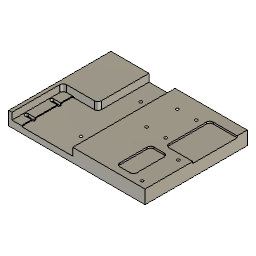
x_stage (Autodesk Fusion 360 design; units mm, degrees)
part number: 2025-09-14-11-39-11-574
Autodesk Fusion 360 part; units mm, degrees
sketch "Sketch1" plane through (0, 0, 0) normal (0, 0, 1) x (1, 0, 0)
  line L0 (-50, 50) -> (50, 50)
  line L1 (50, 50) -> (50, -50)
  line L2 (50, -50) -> (-50, -50)
  line L3 (-50, -50) -> (-50, 50)
  line L4 (-50, 50) -> (50, -50) construction
  line L5 (50, 50) -> (-50, -50) construction
  circle A0 centre (-37.5, 37.5) radius 3.125
  circle A1 centre (-37.5, -37.5) radius 3.125
  circle A2 centre (37.5, -37.5) radius 3.125
  circle A3 centre (37.5, 37.5) radius 3.125
  dimension "d1" = 100
  dimension "d2" = 100
  dimension "d5" = 6.25
  dimension "d6" = 75
  dimension "d7" = 75
  constraint horizontal L0
  constraint perpendicular L0 L1
  constraint parallel L0 L2
  constraint parallel L1 L3
  constraint coincident L4 origin
  constraint coincident L5 origin
  constraint vertical A2.centre A3.centre
  constraint horizontal A0.centre A3.centre
  constraint vertical A0.centre A1.centre
  constraint horizontal A1.centre A2.centre
  constraint equal A2 A3
  constraint equal A1 A2
  constraint equal A0 A1
  constraint coincident L5 A1.centre
  constraint coincident L4 A0.centre
  measures "d1" distance of L0.start L0.end
  measures "d2" distance of L0.start L2.end
  measures "d5" diameter of A0
  measures "d6" distance of A0.centre A3.centre
  measures "d7" distance of A0.centre A1.centre
extrude "Extrude2" add sketch "Sketch1" along normal blind 8
sketch "Sketch2" plane through (0, 0, 8) normal (0, 0, 1) x (-1, 0, 0)
  circle A0 centre (-37.5, -37.5) radius 3.125
  circle A1 centre (37.5, -37.5) radius 3.125
  circle A2 centre (-37.5, 37.5) radius 3.125
  circle A3 centre (37.5, 37.5) radius 3.125
  line L0 (50, 50) -> (-50, 50)
  line L1 (-50, 50) -> (-50, -50)
  line L2 (-50, -50) -> (50, -50)
  line L3 (50, -50) -> (50, 50)
  line L4 (30, -30) -> (-30, -30) construction
  line L5 (-30, -30) -> (-30, 30) construction
  line L6 (-30, 30) -> (30, 30) construction
  line L7 (30, 30) -> (30, -30) construction
  line L8 (30, -30) -> (-30, 30) construction
  line L9 (-30, -30) -> (30, 30) construction
  line L10 (-7.6, -41) -> (7.6, -41)
  line L11 (7.6, -41) -> (7.6, 41)
  line L12 (7.6, 41) -> (-7.6, 41)
  line L13 (-7.6, 41) -> (-7.6, -41)
  line L14 (7.6, 30) -> (28, 30)
  line L15 (28, 30) -> (28, 0)
  line L16 (28, 0) -> (7.6, 0)
  line L17 (7.6, 0) -> (7.6, 30)
  line L18 (28, 30) -> (22.5, 30)
  line L19 (22.5, 30) -> (22.5, 50)
  line L20 (22.5, 50) -> (28, 50)
  line L21 (28, 50) -> (28, 30)
  dimension "d12" = 60
  dimension "d13" = 60
  dimension "d14" = 22.4
  dimension "d15" = 15.2
  dimension "d16" = 11
  dimension "d17" = 11
  dimension "d18" = 30
  dimension "d19" = 20.4
  dimension "d20" = 5.5
  constraint horizontal L4
  constraint perpendicular L4 L5
  constraint parallel L4 L6
  constraint parallel L5 L7
  constraint coincident L8 origin
  constraint coincident L9 origin
  constraint horizontal L10
  constraint vertical L11
  constraint horizontal L12
  constraint vertical L13
  constraint horizontal L14
  constraint vertical L15
  constraint horizontal L16
  constraint vertical L17
  constraint coincident L11 L14.start
  constraint coincident L6 L14.start
  constraint horizontal L18
  constraint vertical L19
  constraint horizontal L20
  constraint vertical L21
  constraint coincident L0 L19.end
  measures "d12" distance of L4.start L4.end
  measures "d13" distance of L4.start L6.end
  measures "d14" distance of L5 L13
  measures "d15" distance of L10.start L10.end
  measures "d16" distance of L4 L10
  measures "d17" distance of L6 L12
  measures "d18" distance of L14.end L15.end
  measures "d19" distance of L15.end L16.end
  measures "d20" distance of L19 L21
extrude "Extrude3" cut sketch "Sketch2" against normal blind 4.5 contours L0 L14 L18 L19 L20 L21 | L11 L14 L15 L16 L17 L18 | L10 L11 L12 L13 L17
fillet "Fillet1" radius 2 7 edges at (-7.6, -30, 5.75) (-7.6, -41, 5.75) (7.6, -41, 5.75) (7.6, 41, 5.75) (-7.6, 41, 5.75) (-7.6, 0, 5.75) (-28, 0, 5.75)
sketch "Sketch3" plane through (0, 0, 8) normal (0, 0, 1) x (-1, 0, 0)
  circle A0 centre (37.5, 37.5) radius 3.125
  circle A1 centre (-37.5, 37.5) radius 3.125
  circle A2 centre (37.5, -37.5) radius 3.125
  circle A3 centre (-37.5, -37.5) radius 3.125
  line L0 (22.5, 30) -> (22.5, 50)
  line L1 (22.5, 50) -> (-50, 50)
  line L2 (-50, 50) -> (-50, -50)
  line L3 (50, -50) -> (50, 50)
  line L4 (50, 50) -> (28, 50)
  line L5 (28, 50) -> (28, 2)
  arc A4 (26, 0) -> (28, 2) centre (26, 2) ccw
  line L6 (26, 0) -> (9.6, 0)
  arc A5 (9.6, 0) -> (7.6, -2) centre (9.6, -2) ccw
  line L7 (7.6, -2) -> (7.6, -39)
  arc A6 (5.6, -41) -> (7.6, -39) centre (5.6, -39) ccw
  arc A7 (-5.6, 41) -> (-7.6, 39) centre (-5.6, 39) ccw
  line L8 (-5.6, 41) -> (5.6, 41)
  arc A8 (7.6, 39) -> (5.6, 41) centre (5.6, 39) ccw
  line L9 (7.6, 39) -> (7.6, 32)
  arc A9 (7.6, 32) -> (9.6, 30) centre (9.6, 32) ccw
  line L10 (9.6, 30) -> (22.5, 30)
  circle A10 centre (0, -17.5) radius 1.5
  circle A11 centre (0, 17.5) radius 1.5
  circle A12 centre (-19, -2) radius 1.5
  circle A13 centre (-30, -2) radius 1.5
  circle A14 centre (-30, -20) radius 1.5
  circle A15 centre (-19, -20) radius 1.5
  line L11 (26.5, 9) -> (22.5, 9)
  arc A16 (22.5, 9) -> (22.5, 7) centre (22.5, 8) ccw
  line L12 (22.5, 7) -> (26.5, 7)
  arc A17 (26.5, 7) -> (26.5, 9) centre (26.5, 8) ccw
  line L13 (26.5, 8) -> (22.5, 8) construction
  line L14 (26.5, 24) -> (22.5, 24)
  arc A18 (22.5, 24) -> (22.5, 22) centre (22.5, 23) ccw
  line L15 (22.5, 22) -> (26.5, 22)
  arc A19 (26.5, 22) -> (26.5, 24) centre (26.5, 23) ccw
  line L16 (26.5, 23) -> (22.5, 23) construction
  line L17 (-30, -30) -> (-30, 30)
  line L18 (30, -30) -> (-30, -30)
  line L19 (30, 30) -> (30, -30)
  line L20 (-30, 30) -> (30, 30)
  circle A20 centre (-45, 5.5) radius 1.5
  circle A21 centre (-45, 26.7) radius 1.5
  line L21 (-50, -50) -> (50, -50)
  line L22 (-7.6, -39) -> (-7.6, 39)
  dimension "d27" = 3
  dimension "d28" = 3
  dimension "d29" = 1
  dimension "d30" = 4
  dimension "d32" = 15
  dimension "d33" = 7
  dimension "d34" = 35
  dimension "d35" = 17.5
  dimension "d36" = 11
  dimension "d37" = 18
  dimension "d43" = 30
  dimension "d48" = 7.5
  dimension "d94" = 21.2
  dimension "d95" = 3
  dimension "d96" = 100
  dimension "d98" = 5
  dimension "d122" = 30
  dimension "d123" = 7.5
  dimension "d141" = 69
  constraint tangent L11 A16
  constraint tangent A16 L12
  constraint parallel L11 L12
  constraint tangent L12 A17
  constraint tangent L11 A17
  constraint horizontal L13
  constraint tangent L14 A18
  constraint tangent A18 L15
  constraint parallel L14 L15
  constraint tangent L15 A19
  constraint tangent L14 A19
  constraint horizontal L16
  constraint equal A10 A11
  constraint equal A12 A13
  constraint equal A12 A15
  constraint equal A14 A15
  constraint horizontal A14.centre A15.centre
  constraint vertical A13.centre A14.centre
  constraint horizontal A12.centre A13.centre
  constraint vertical A12.centre A15.centre
  constraint vertical A10.centre A11.centre
  constraint vertical A16.centre A18.centre
  constraint vertical A17.centre A19.centre
  constraint equal A16 A18
  constraint vertical origin A11.centre
  constraint vertical A20.centre A21.centre
  constraint equal A20 A21
  measures "d27" diameter of A11
  measures "d28" diameter of A12
  measures "d29" radius of A17
  measures "d30" distance of A18.end L15.end
  measures "d32" distance of A17.centre A19.centre
  measures "d33" distance of L10 A18.centre
  measures "d34" distance of A10.centre A11.centre
  measures "d35" distance of origin A10.centre
  measures "d36" distance of A12.centre A13.centre
  measures "d37" distance of A12.centre A15.centre
  measures "d43" distance of L6 L18
  measures "d48" distance of A16.centre L19
  measures "d94" distance of A20.centre A21.centre
  measures "d95" diameter of A20
  measures "d96" distance of L3.start L3.end
  measures "d98" distance of L2 A20.centre
  measures "d122" distance of A14.centre L21
  measures "d123" vertical distance of A13.centre A20.centre
  measures "d141" distance of L3 A15.centre
sketch "Sketch4" plane through (0, 0, 3.5) normal (0, 0, 1) x (-1, 0, 0)
  arc A0 (5.6, -41) -> (7.6, -39) centre (5.6, -39) ccw
  line L0 (7.6, -39) -> (7.6, -2)
  arc A1 (9.6, 0) -> (7.6, -2) centre (9.6, -2) ccw
  line L1 (9.6, 0) -> (26, 0)
  arc A2 (26, 0) -> (28, 2) centre (26, 2) ccw
  line L2 (28, 2) -> (28, 50)
  line L3 (28, 50) -> (22.5, 50)
  line L4 (22.5, 50) -> (22.5, 30)
  line L5 (22.5, 30) -> (9.6, 30)
  arc A3 (7.6, 32) -> (9.6, 30) centre (9.6, 32) ccw
  line L6 (7.6, 32) -> (7.6, 39)
  arc A4 (7.6, 39) -> (5.6, 41) centre (5.6, 39) ccw
  line L7 (5.6, 41) -> (-5.6, 41)
  arc A5 (-5.6, 41) -> (-7.6, 39) centre (-5.6, 39) ccw
  line L8 (-7.6, 39) -> (-7.6, -39)
  arc A6 (-7.6, -39) -> (-5.6, -41) centre (-5.6, -39) ccw
  line L9 (-5.6, -41) -> (5.6, -41)
  line L10 (28, 50) -> (22.5, 50)
  line L11 (22.5, 50) -> (22.5, 0)
  line L12 (22.5, 0) -> (28, 0)
  line L13 (28, 0) -> (28, 50)
  line L14 (22.5, 30) -> (22.5, 50)
  dimension "d47" = 50
  constraint horizontal L10
  constraint vertical L11
  constraint horizontal L12
  constraint vertical L13
  constraint coincident L2.end L3.start
  constraint collinear L11 L14
  measures "d47" distance of L3.end L11.end
extrude "Extrude4" add sketch "Sketch4" along normal blind 0.5 contours L1 A2 L2 L3 L4 L10 L11 L12 L13 L14
extrude "Extrude5" cut sketch "Sketch3" against normal up to surface (8 mm away) contours A0 | A1 | A2 | A3 | A13 L17 | A13 L17 | A14 L17 | A14 L17 | A10 | A11 | A12 | A15 | L11 A16 L12 A17 | L14 A18 L15 A19 | A20 | A21
sketch "Sketch5" plane through (0, 0, 8) normal (0, 0, 1) x (-1, 0, 0)
  circle A0 centre (-30, -2) radius 1.5
  circle A1 centre (-30, -20) radius 1.5
  line L0 (28, 50) -> (28, 2)
  arc A2 (26, 0) -> (28, 2) centre (26, 2) ccw
  line L1 (26, 0) -> (9.6, 0)
  arc A3 (9.6, 0) -> (7.6, -2) centre (9.6, -2) ccw
  line L2 (7.6, -2) -> (7.6, -39)
  circle A4 centre (-37.5, 37.5) radius 5.5
  circle A5 centre (-37.5, -37.5) radius 5.5
  circle A6 centre (37.5, -37.5) radius 5.5
  circle A7 centre (37.5, 37.5) radius 5.5
  circle A8 centre (-45, 5.5) radius 1.5
  circle A9 centre (-19, -20) radius 1.5
  circle A10 centre (-19, -2) radius 1.5
  circle A11 centre (-45, 26.7) radius 1.5
  arc A12 (5.6, -41) -> (7.6, -39) centre (5.6, -39) ccw
  line L3 (5.6, -41) -> (-5.6, -41)
  arc A13 (-7.6, -39) -> (-5.6, -41) centre (-5.6, -39) ccw
  line L4 (-7.6, -39) -> (-7.6, 39)
  arc A14 (-5.6, 41) -> (-7.6, 39) centre (-5.6, 39) ccw
  line L5 (-5.6, 41) -> (5.6, 41)
  arc A15 (7.6, 39) -> (5.6, 41) centre (5.6, 39) ccw
  line L6 (7.6, 39) -> (7.6, 32)
  arc A16 (7.6, 32) -> (9.6, 30) centre (9.6, 32) ccw
  line L7 (9.6, 30) -> (22.5, 30)
  line L8 (22.5, 30) -> (22.5, 50)
  line L9 (22.5, 50) -> (-50, 50)
  line L10 (-50, 50) -> (-50, -50)
  line L11 (-50, -50) -> (50, -50)
  line L12 (50, -50) -> (50, 50)
  line L13 (50, 50) -> (28, 50)
  circle A17 centre (-37.5, -37.5) radius 3.125
  circle A18 centre (37.5, -37.5) radius 3.125
  circle A19 centre (-37.5, 37.5) radius 3.125
  circle A20 centre (37.5, 37.5) radius 3.125
  dimension "d69" = 11
  constraint equal A5 A6
  constraint equal A4 A5
  constraint equal A4 A7
  constraint coincident A5.centre A17.centre
  constraint coincident A6.centre A18.centre
  constraint coincident A7.centre A20.centre
  constraint coincident A4.centre A19.centre
  measures "d69" diameter of A7
extrude "Extrude6" cut sketch "Sketch5" against normal blind 6 contours A4 | A5 | A6 | A7 | A17 | A18 | A19 | A20
fillet "Fillet2" radius 1 2 edges at (-22.5, -30, 3.75) (-22.5, 0, 3.75)
fillet "Fillet3" radius 2 1 edges at (-22.5, -30, 6)
sketch "Sketch6" plane through (0, 0, 0) normal (0, 0, -1) x (1, 0, 0)
  circle A0 centre (0, 17.5) radius 1.5
  line L0 (-22.5, 22) -> (-26.5, 22)
  arc A1 (-26.5, 24) -> (-26.5, 22) centre (-26.5, 23) ccw
  line L1 (-26.5, 24) -> (-22.5, 24)
  arc A2 (-22.5, 22) -> (-22.5, 24) centre (-22.5, 23) ccw
  circle A3 centre (30, -2) radius 1.5
  circle A4 centre (0, -17.5) radius 1.5
  line L2 (-22.5, 7) -> (-26.5, 7)
  arc A5 (-26.5, 9) -> (-26.5, 7) centre (-26.5, 8) ccw
  line L3 (-26.5, 9) -> (-22.5, 9)
  arc A6 (-22.5, 7) -> (-22.5, 9) centre (-22.5, 8) ccw
  circle A7 centre (30, -20) radius 1.5
  line L4 (50, 50) -> (-50, 50)
  line L5 (-26.5, 21) -> (-22.5, 21)
  arc A8 (-22.5, 21) -> (-22.5, 25) centre (-22.5, 23) ccw
  line L6 (-22.5, 25) -> (-26.5, 25)
  arc A9 (-26.5, 25) -> (-26.5, 21) centre (-26.5, 23) ccw
  line L7 (-26.5, 23) -> (-22.5, 23) construction
  line L8 (-26.5, 6) -> (-22.5, 6)
  arc A10 (-22.5, 6) -> (-22.5, 10) centre (-22.5, 8) ccw
  line L9 (-22.5, 10) -> (-26.5, 10)
  arc A11 (-26.5, 10) -> (-26.5, 6) centre (-26.5, 8) ccw
  line L10 (-26.5, 8) -> (-22.5, 8) construction
  circle A12 centre (45, 5.5) radius 1.5
  circle A13 centre (19, -20) radius 1.5
  circle A14 centre (19, -2) radius 1.5
  circle A15 centre (45, 26.7) radius 1.5
  circle A16 centre (37.5, -37.5) radius 3.125
  circle A17 centre (-37.5, -37.5) radius 3.125
  circle A18 centre (37.5, 37.5) radius 3.125
  circle A19 centre (-37.5, 37.5) radius 3.125
  line L11 (-50, 50) -> (-50, -50)
  line L12 (-50, -50) -> (50, -50)
  line L13 (50, -50) -> (50, 50)
  dimension "d76" = 2
  dimension "d77" = 2
  constraint tangent L5 A8
  constraint tangent A8 L6
  constraint parallel L5 L6
  constraint tangent L6 A9
  constraint tangent L5 A9
  constraint coincident A2.centre A8.centre
  constraint horizontal L7
  constraint coincident A1.centre A9.centre
  constraint tangent L8 A10
  constraint tangent A10 L9
  constraint parallel L8 L9
  constraint tangent L9 A11
  constraint tangent L8 A11
  constraint coincident A6.centre A10.centre
  constraint horizontal L10
  constraint coincident A5.centre A11.centre
  measures "d76" radius of A10
  measures "d77" radius of A8
extrude "Extrude7" cut sketch "Sketch6" against normal blind 2.5 contours L5 A8 L6 A9 | L8 A10 L9 A11
sketch "Sketch7" plane through (0, 0, 8) normal (0, 0, 1) x (-1, 0, 0)
  line L0 (28, 50) -> (28, 2)
  arc A0 (26, 0) -> (28, 2) centre (26, 2) ccw
  line L1 (7.6, -2) -> (7.6, -39)
  circle A1 centre (-30, -2) radius 1.5
  circle A2 centre (-30, -20) radius 1.5
  line L2 (-17, -22) -> (-45, -22)
  line L3 (-45, 0) -> (-17, 0)
  arc A3 (20.5, 30) -> (22.5, 32) centre (20.5, 32) ccw
  line L4 (22.5, 32) -> (22.5, 50)
  line L5 (22.5, 50) -> (-50, 50)
  line L6 (-50, 50) -> (-50, -50)
  line L7 (-50, -50) -> (50, -50)
  line L8 (50, -50) -> (50, 50)
  line L9 (50, 50) -> (28, 50)
  arc A4 (5.6, -41) -> (7.6, -39) centre (5.6, -39) ccw
  line L10 (5.6, -41) -> (-5.6, -41)
  arc A5 (-7.6, -39) -> (-5.6, -41) centre (-5.6, -39) ccw
  line L11 (-7.6, -39) -> (-7.6, 39)
  arc A6 (-5.6, 41) -> (-7.6, 39) centre (-5.6, 39) ccw
  line L12 (-5.6, 41) -> (5.6, 41)
  arc A7 (7.6, 39) -> (5.6, 41) centre (5.6, 39) ccw
  line L13 (7.6, 39) -> (7.6, 32)
  arc A8 (7.6, 32) -> (9.6, 30) centre (9.6, 32) ccw
  line L14 (9.6, 30) -> (20.5, 30)
  circle A9 centre (37.5, -37.5) radius 5.5
  circle A10 centre (37.5, 37.5) radius 5.5
  circle A11 centre (-37.5, -37.5) radius 5.5
  circle A12 centre (-37.5, 37.5) radius 5.5
  circle A13 centre (-45, 5.5) radius 1.5
  circle A14 centre (-19, -20) radius 1.5
  circle A15 centre (-19, -2) radius 1.5
  circle A16 centre (-45, 26.7) radius 1.5
  line L15 (-50, -24) -> (-34, -24)
  line L16 (-34, -24) -> (-34, 2)
  line L17 (-34, 2) -> (-50, 2)
  line L18 (-50, 2) -> (-50, -24)
  line L19 (-29.3, 29.75) -> (-55.5, 29.75)
  line L20 (-55.5, 2.45) -> (-29.3, 2.45)
  line L21 (-29.3, 2.45) -> (-29.3, 29.75)
  line L22 (-29.3, 6.1) -> (-39.3, 6.1)
  line L23 (-39.3, 6.1) -> (-39.3, 26.1)
  line L24 (-39.3, 26.1) -> (-29.3, 26.1)
  line L25 (-29.3, 26.1) -> (-29.3, 6.1)
  dimension "d106" = 2
  dimension "d107" = 2
  dimension "d108" = 16
  dimension "d115" = 20
  dimension "d116" = 27.3
  dimension "d117" = 3.65
  dimension "d118" = 10
  constraint horizontal L15
  constraint vertical L16
  constraint horizontal L17
  constraint vertical L18
  constraint coincident L6 L15.start
  constraint horizontal L22
  constraint vertical L23
  constraint horizontal L24
  constraint vertical L25
  constraint coincident L21 L22.start
  measures "d106" distance of L2 L15
  measures "d107" distance of L3 L17
  measures "d108" distance of L15.start L15.end
  measures "d115" distance of L22.end L23.end
  measures "d116" distance of L20.end L19.start
  measures "d117" distance of L20 L22
  measures "d118" distance of L22.start L22.end
extrude "Extrude9" cut sketch "Sketch7" against normal blind 1 contours L6 L15 L16 L17 L18 | L21 L22 L23 L24 L25
fillet "Fillet6" radius 2 6 edges at (29.3, -6.1, 7.5) (29.3, -26.1, 7.5) (39.3, -26.1, 7.5) (39.3, -6.1, 7.5) (34, -2, 7.5) (34, 24, 7.5)
thread "Thread1" "ISO Metric profile 2.0 M2x0.4 M2x0.4 6H" major diameter 2.074 minor diameter 1.623 pitch 0.4 angle 60 resizes the face on face at (-1.4925, -17.3506, 2.3333) on face at (-1.4925, 17.6494, 2.3333) on face at (28.5075, 19.8506, 5.3333) on face at (17.5075, 2.1494, 2.6667) on face at (20.4925, 20.1494, 2.6667) on face at (28.5075, 1.8506, 5.3333) on face at (45.6843, -25.3652, 5.3333) on face at (45.6843, -4.1652, 5.3333)
sketch "Sketch9" plane through (0, 0, 0) normal (0, 0, -1) x (1, 0, 0)
  line L0 (-22.5, 21) -> (-26.5, 21)
  arc A0 (-26.5, 25) -> (-26.5, 21) centre (-26.5, 23) ccw
  line L1 (-26.5, 25) -> (-22.5, 25)
  arc A1 (-22.5, 21) -> (-22.5, 25) centre (-22.5, 23) ccw
  line L2 (-22.5, 6) -> (-26.5, 6)
  arc A2 (-26.5, 10) -> (-26.5, 6) centre (-26.5, 8) ccw
  line L3 (-26.5, 10) -> (-22.5, 10)
  arc A3 (-22.5, 6) -> (-22.5, 10) centre (-22.5, 8) ccw
  circle A4 centre (30, -20) radius 0.8115
  circle A5 centre (0, -17.5) radius 0.8115
  circle A6 centre (30, -2) radius 0.8115
  circle A7 centre (45, 5.5) radius 0.8115
  circle A8 centre (19, -20) radius 0.8115
  circle A9 centre (0, 17.5) radius 0.8115
  circle A10 centre (19, -2) radius 0.8115
  circle A11 centre (45, 26.7) radius 0.8115
  circle A12 centre (-37.5, -37.5) radius 3.125
  circle A13 centre (37.5, 37.5) radius 3.125
  circle A14 centre (-37.5, 37.5) radius 3.125
  circle A15 centre (37.5, -37.5) radius 3.125
  line L4 (50, 50) -> (-50, 50)
  line L5 (-50, 50) -> (-50, -50)
  line L6 (-50, -50) -> (50, -50)
  line L7 (50, -50) -> (50, 50)
  line L8 (-30, 30) -> (30, 30)
  line L9 (30, 30) -> (30, -30)
  line L10 (30, -30) -> (-30, -30)
  line L11 (-30, -30) -> (-30, 30)
  line L12 (-30, 30) -> (30, -30) construction
  line L13 (30, 30) -> (-30, -30) construction
  line L14 (30, 30) -> (50, 30)
  line L15 (50, 30) -> (50, -30)
  line L16 (50, -30) -> (30, -30)
  line L17 (30, -30) -> (30, 30)
  dimension "d136" = 60
  dimension "d137" = 60
  dimension "d140" = 20
  constraint horizontal L8
  constraint perpendicular L8 L9
  constraint parallel L8 L10
  constraint parallel L9 L11
  constraint coincident L12 origin
  constraint coincident L13 origin
  constraint horizontal L14
  constraint vertical L15
  constraint horizontal L16
  constraint vertical L17
  constraint collinear L10 L16
  measures "d136" distance of L8.start L8.end
  measures "d137" distance of L8.start L10.end
  measures "d140" distance of L15 L17
extrude "Extrude11" cut sketch "Sketch9" against normal up to surface (8 mm away) contours L4 L5 L6 L7 L8 L10 L11 L14 L16
sketch "Sketch8" plane through (0, 0, 8) normal (0, 0, 1) x (-1, 0, 0)
  circle A0 centre (-45, 27.2) radius 1.5
  circle A1 centre (-19, -2) radius 1.5
  circle A2 centre (-19, -20) radius 1.5
  circle A3 centre (-45, 6) radius 1.5
  circle A4 centre (-30, -2) radius 1.5
  circle A5 centre (-30, -20) radius 1.5
  circle A6 centre (-37.5, 37.5) radius 5.5
  circle A7 centre (-37.5, -37.5) radius 5.5
  circle A8 centre (37.5, 37.5) radius 5.5
  circle A9 centre (37.5, -37.5) radius 5.5
  line L0 (-50, 2) -> (-36, 2)
  arc A10 (-34, 0) -> (-36, 2) centre (-36, 0) ccw
  line L1 (-34, 0) -> (-34, -22)
  arc A11 (-36, -24) -> (-34, -22) centre (-36, -22) ccw
  line L2 (-36, -24) -> (-50, -24)
  line L3 (-50, -24) -> (-50, -50)
  line L4 (-50, -50) -> (50, -50)
  line L5 (50, -50) -> (50, 50)
  line L6 (50, 50) -> (28, 50)
  line L7 (28, 50) -> (28, 2)
  arc A12 (26, 0) -> (28, 2) centre (26, 2) ccw
  line L8 (26, 0) -> (9.6, 0)
  arc A13 (9.6, 0) -> (7.6, -2) centre (9.6, -2) ccw
  line L9 (7.6, -2) -> (7.6, -39)
  arc A14 (5.6, -41) -> (7.6, -39) centre (5.6, -39) ccw
  line L10 (5.6, -41) -> (-5.6, -41)
  arc A15 (-7.6, -39) -> (-5.6, -41) centre (-5.6, -39) ccw
  line L11 (-7.6, -39) -> (-7.6, 39)
  arc A16 (-5.6, 41) -> (-7.6, 39) centre (-5.6, 39) ccw
  line L12 (-5.6, 41) -> (5.6, 41)
  arc A17 (7.6, 39) -> (5.6, 41) centre (5.6, 39) ccw
  line L13 (7.6, 39) -> (7.6, 32)
  arc A18 (7.6, 32) -> (9.6, 30) centre (9.6, 32) ccw
  line L14 (9.6, 30) -> (20, 30)
  arc A19 (20, 30) -> (22, 32) centre (20, 32) ccw
  line L15 (22, 32) -> (22, 50)
  line L16 (22, 50) -> (-50, 50)
  line L17 (-50, 50) -> (-50, 2)
  line L18 (-39.3, 8.6) -> (-39.3, 24.6)
  arc A20 (-37.3, 26.6) -> (-39.3, 24.6) centre (-37.3, 24.6) ccw
  line L19 (-37.3, 26.6) -> (-31.3, 26.6)
  arc A21 (-29.3, 24.6) -> (-31.3, 26.6) centre (-31.3, 24.6) ccw
  line L20 (-29.3, 24.6) -> (-29.3, 8.6)
  arc A22 (-31.3, 6.6) -> (-29.3, 8.6) centre (-31.3, 8.6) ccw
  line L21 (-31.3, 6.6) -> (-37.3, 6.6)
  arc A23 (-39.3, 8.6) -> (-37.3, 6.6) centre (-37.3, 8.6) ccw
  line L22 (-45, -22) -> (-17, -22)
  line L23 (-17, -22) -> (-17, 0)
  line L24 (-17, 0) -> (-45, 0)
  line L25 (-17, -23.5) -> (-37, -23.5)
  line L26 (-37, -23.5) -> (-37, 1.5)
  line L27 (-37, 1.5) -> (-17, 1.5)
  line L28 (-17, 1.5) -> (-17, -23.5)
  line L29 (-17, -23.5) -> (-15.85, -23.5)
  line L30 (-15.85, -23.5) -> (-15.85, 1.5)
  line L31 (-15.85, 1.5) -> (-17, 1.5)
  line L32 (-17, 1.5) -> (-17, -23.5)
  dimension "d124" = 1.5
  dimension "d125" = 1.5
  dimension "d126" = 20
  dimension "d131" = 1.15
  constraint horizontal L25
  constraint vertical L26
  constraint horizontal L27
  constraint vertical L28
  constraint collinear L23 L28
  constraint horizontal L29
  constraint vertical L30
  constraint horizontal L31
  constraint vertical L32
  constraint collinear L27 L31
  measures "d124" distance of L22 L25
  measures "d125" distance of L24 L27
  measures "d126" distance of L25.start L25.end
  measures "d131" distance of L25.start L29.end
extrude "Extrude10" [suppressed]
fillet "Fillet8" [suppressed]
equation "d2 = d1"
equation "d7 = d6"
equation "d13 = d12"
equation "d17 = d16"
equation "d28 = d27"
equation "d35 = d34 / 2"
equation "d77 = d76"
equation "d95 = d28"
equation "d107 = d106"
equation "d117 = ( d116 - d115 ) / 2"
equation "d125 = d124"
equation "d131 = 1.85 mm - 0.7 mm"
equation "d137 = d136"
